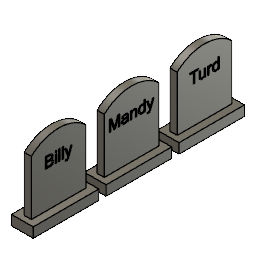
Nick Tomb Stones v2 (Autodesk Fusion 360 design; units mm, degrees)
Autodesk Fusion 360 part; units mm, degrees
note: some values were not read from the file. Set by a fixed rule: which face or edge a step refers to.
sketch "Sketch1" plane through (0, 0, 0) normal (1, 0, 0) x (0, 0, -1)
  line L0 (0, 0) -> (30, 0)
  line L1 (30, 0) -> (30, 36)
  line L2 (30, 36) -> (0, 36)
  line L3 (0, 36) -> (0, 0)
  line L4 (0, 36) -> (0, 30)
  line L5 (30, 36) -> (30, 30)
  arc A0 (30, 30) -> (0, 30) centre (15, 14.25) ccw
  dimension "d1" = 30
  dimension "d2" = 36
  dimension "d3" = 6
  dimension "d4" = 6
  constraint horizontal L0
  constraint vertical L1
  constraint horizontal L2
  constraint vertical L3
  constraint coincident L0.start L3.end
  constraint perpendicular L2 L4
  constraint perpendicular L2 L5
  constraint tangent L2 A0
  measures "d1" distance of L0.start L0.end
  measures "d2" distance of L0.start L2.end
  measures "d3" distance of L2.end L4.end
  measures "d4" distance of L1.end L5.end
extrude "Extrude1" add sketch "Sketch1" along normal blind 4 contours L0 L1 L3 A0 makes body 1
sketch "Sketch2" plane through (0, 0, 0) normal (0, -1, 0) x (1, 0, 0)
  line L0 (0, 0) -> (0, -30)
  line L1 (0, -30) -> (4, -30)
  line L2 (4, -30) -> (4, 0)
  line L3 (4, 0) -> (0, 0)
  line L4 (4, -15) -> (4, 3)
  line L5 (2, 0) -> (8, 0)
  line L6 (8, 3) -> (-4, 3)
  line L7 (-4, 3) -> (-4, -33)
  line L8 (-4, -33) -> (8, -33)
  line L9 (8, -33) -> (8, 3)
  dimension "d7" = 18
  dimension "d8" = 6
  dimension "d9" = 12
  dimension "d10" = 36
  constraint midpoint L2 L4.start
  constraint perpendicular L3 L4
  constraint midpoint L3 L5.start
  constraint perpendicular L0 L5
  constraint horizontal L6
  constraint vertical L7
  constraint horizontal L8
  constraint vertical L9
  measures "d7" distance of L4.start L4.end
  measures "d8" distance of L5.start L5.end
  measures "d9" distance of L6.start L6.end
  measures "d10" distance of L6.start L8.end
extrude "Extrude2" add sketch "Sketch2" along normal blind 6 separate body makes body 2
extrude "Extrude3" add 1 faces at (1.3333, 0, -10) along direction (0, -1, 0) blind 6 on bodies 1 bodies 1 2
sketch "Sketch3" plane through (4, 0, 0) normal (1, 0, 0) x (0, 0, -1)
  arc A0 (30, 30) -> (0, 30) centre (15, 14.25) ccw
  line L0 (0, 30) -> (0, 0)
  line L1 (0, 0) -> (30, 0)
  line L2 (30, 0) -> (30, 30)
  line L3 (0, 30) -> (2, 30)
  line L4 (2, 30) -> (2, 28)
  line L5 (2, 28) -> (0, 28)
  line L6 (0, 28) -> (0, 30)
  line L7 (2, 28) -> (28, 28)
  line L8 (28, 28) -> (28, 18)
  line L9 (28, 18) -> (2, 18)
  line L10 (2, 18) -> (2, 28)
  line L11 (2, 18) -> (28, 18) construction
  line L12 (28, 18) -> (28, 28) construction
  line L13 (28, 28) -> (2, 28) construction
  line L14 (2, 28) -> (2, 18) construction
  dimension "d15" = 2
  dimension "d16" = 2
  dimension "d17" = 26
  dimension "d18" = 10
  dimension "d19" = 6
  text T0 "Billy" font "Arial" height 6 align centre middle in box 26 x 10 at (2, 18) x (1, 0) y (0, 1) spacing 1 kerned
  constraint horizontal L3
  constraint vertical L4
  constraint horizontal L5
  constraint vertical L6
  constraint coincident A0.end L0.start
  constraint horizontal L7
  constraint vertical L8
  constraint horizontal L9
  constraint vertical L10
  constraint coincident L8.end
  constraint coincident L4.end
  measures "d15" distance of A0.end L3.end
  measures "d16" distance of A0.end L5.end
  measures "d17" distance of L4.end L7.end
  measures "d18" distance of L4.end L9.end
extrude "Extrude4" cut sketch "Sketch3" against normal blind 1 text T0 bodies 1
sketch "Sketch4" plane through (0, -6, 0) normal (0, -1, 0) x (1, 0, 0)
  line L0 (8, -33) -> (8, 3)
  line L1 (8, 3) -> (-4, 3)
  line L2 (-4, 3) -> (-4, -33)
  line L3 (-4, -33) -> (8, -33)
  line L4 (2, 3) -> (2, -33)
  line L5 (6.75, -12.2576) -> (2, -9.5152)
  line L6 (2, -9.5152) -> (-2.75, -12.2576)
  line L7 (-2.75, -12.2576) -> (-2.75, -17.7424)
  line L8 (-2.75, -17.7424) -> (2, -20.4848)
  line L9 (2, -20.4848) -> (6.75, -17.7424)
  line L10 (6.75, -17.7424) -> (6.75, -12.2576)
  point P0 (2, -15)
  dimension "d22" = 4.75
  constraint midpoint L1 L4.start
  constraint midpoint L3 L4.end
  constraint midpoint L4 P0
  measures "d22" distance of P0 L10
extrude "Extrude5" cut sketch "Sketch4" against normal blind 3.3 contours L4 L6 L7 L8 | L4 L5 L9 L10 bodies 1
sketch "Sketch5" plane through (0, -6, 0) normal (0, -1, 0) x (1, 0, 0)
  line L0 (2, -9.5152) -> (6.75, -12.2576)
  line L1 (6.75, -12.2576) -> (6.75, -17.7424)
  line L2 (6.75, -17.7424) -> (2, -20.4848)
  line L3 (2, -20.4848) -> (-2.75, -17.7424)
  line L4 (-2.75, -17.7424) -> (-2.75, -12.2576)
  line L5 (-2.75, -12.2576) -> (2, -9.5152)
  line L6 (8, -33) -> (8, 3)
  line L7 (8, 3) -> (-4, 3)
  line L8 (-4, 3) -> (-4, -33)
  line L9 (-4, -33) -> (8, -33)
  line L10 (2, -9.5152) -> (2, 3)
  line L11 (2, -20.4848) -> (2, -33)
  line L12 (4.7424, -31.4924) -> (7.4848, -26.7424)
  line L13 (7.4848, -26.7424) -> (4.7424, -21.9924)
  line L14 (4.7424, -21.9924) -> (-0.7424, -21.9924)
  line L15 (-0.7424, -21.9924) -> (-3.4848, -26.7424)
  line L16 (-3.4848, -26.7424) -> (-0.7424, -31.4924)
  line L17 (-0.7424, -31.4924) -> (4.7424, -31.4924)
  line L18 (4.7424, -8.0076) -> (7.4848, -3.2576)
  line L19 (7.4848, -3.2576) -> (4.7424, 1.4924)
  line L20 (4.7424, 1.4924) -> (-0.7424, 1.4924)
  line L21 (-0.7424, 1.4924) -> (-3.4848, -3.2576)
  line L22 (-3.4848, -3.2576) -> (-0.7424, -8.0076)
  line L23 (-0.7424, -8.0076) -> (4.7424, -8.0076)
  point P0 (2, -26.7424)
  point P1 (2, -3.2576)
  dimension "d25" = 4.75
  dimension "d26" = 4.75
  constraint coincident L0.start L5.end
  constraint midpoint L7 L10.end
  constraint coincident L2.end L3.start
  constraint midpoint L9 L11.end
  constraint midpoint L11 P0
  constraint midpoint L10 P1
  measures "d25" distance of P0 L17
  measures "d26" distance of P1 L23
extrude "Extrude6" cut sketch "Sketch5" against normal blind 3.3 contours L10 L20 L21 L22 L23 | L10 L18 L19 L20 L23 | L11 L12 L13 L14 L17 | L11 L14 L15 L16 L17 bodies 1
chamfer "Chamfer1" distance 0.5 angle 45 21 edges at (8, -6, -15) (2, -6, 3) (-4, -6, -15) (2, -6, -33) (6.1136, -6, -24.3674) (6.1136, -6, -29.1174) (2, -6, -31.4924) (-2.1136, -6, -29.1174) (-2.1136, -6, -24.3674) (-0.375, -6, -19.1136) (4.375, -6, -19.1136) (6.75, -6, -15) (4.375, -6, -10.8864) (-0.375, -6, -10.8864) (-2.75, -6, -15) (-2.1136, -6, -5.6326) (2, -6, -8.0076) (6.1136, -6, -5.6326) (6.1136, -6, -0.8826) (2, -6, 1.4924) (-2.1136, -6, -0.8826) on bodies 1
extrude "Extrude7" cut 3 faces at (1.0859, -2.7, -28.3257) (3.5833, -2.7, -15.9141) (1.0859, -2.7, -4.8409) along direction (0, 1, 0) blind 0.5 on bodies 1 bodies 1
copy_body "CopyPasteBodies1" bodies 1 makes body 3
move_body "Move1" bodies 3 to x (1, 0, 0) y (0, 1, 0) z (0, 0, 1) at (0, 0, -40)
extrude "Extrude8" add 6 faces at (3, 22.9236, -47.9243) (3, 21.4488, -53.6842) (3, 25.4352, -53.6842) (3, 22, -55.5259) (3, 22, -57.3881) (3, 22.0559, -59.4741) along direction (1, 0, 0) blind 1 on bodies 3 bodies 3
copy_body "CopyPasteBodies2" bodies 3 makes body 4
move_body "Move2" bodies 4 to x (1, 0, 0) y (0, 1, 0) z (0, 0, 1) at (0, 0, -40)
sketch "Sketch6" plane through (4, 0, 0) normal (1, 0, 0) x (0, 0, -1)
  arc A0 (70, 30) -> (40, 30) centre (55, 14.25) ccw
  line L0 (40, 30) -> (40, 0)
  line L1 (40, 0) -> (70, 0)
  line L2 (70, 0) -> (70, 30)
  line L3 (40, 30) -> (42, 30)
  line L4 (42, 30) -> (42, 28)
  line L5 (42, 28) -> (40, 28)
  line L6 (40, 28) -> (40, 30)
  line L7 (42, 28) -> (68, 28)
  line L8 (68, 28) -> (68, 18)
  line L9 (68, 18) -> (42, 18)
  line L10 (42, 18) -> (42, 28)
  line L11 (42, 18) -> (68, 18) construction
  line L12 (68, 18) -> (68, 28) construction
  line L13 (68, 28) -> (42, 28) construction
  line L14 (42, 28) -> (42, 18) construction
  dimension "d34" = 2
  dimension "d35" = 2
  dimension "d36" = 26
  dimension "d37" = 10
  dimension "d38" = 6
  text T0 "Mandy" font "Arial" height 6 align centre middle in box 26 x 10 at (42, 18) x (1, 0) y (0, 1) spacing 1 kerned
  constraint horizontal L3
  constraint vertical L4
  constraint horizontal L5
  constraint vertical L6
  constraint coincident A0.end L0.start
  constraint horizontal L7
  constraint vertical L8
  constraint horizontal L9
  constraint vertical L10
  constraint coincident L8.end
  constraint coincident L4.end
  measures "d34" distance of A0.end L3.end
  measures "d35" distance of A0.end L5.end
  measures "d36" distance of L4.end L7.end
  measures "d37" distance of L4.end L9.end
extrude "Extrude9" cut sketch "Sketch6" against normal blind 0.5 text T0 bodies 3
extrude "Extrude10" add 6 faces at (3, 22.9236, -7.9243) (3, 21.4488, -13.6842) (3, 25.4352, -13.6842) (3, 22, -15.5259) (3, 22, -17.3881) (3, 22.0559, -19.4741) along direction (1, 0, 0) blind 0.5 on bodies 1 bodies 1
sketch "Sketch7" plane through (4, 0, 0) normal (1, 0, 0) x (0, 0, -1)
  arc A0 (110, 30) -> (80, 30) centre (95, 14.25) ccw
  line L0 (80, 30) -> (80, 0)
  line L1 (80, 0) -> (110, 0)
  line L2 (110, 0) -> (110, 30)
  line L3 (80, 30) -> (82, 30)
  line L4 (82, 30) -> (82, 28)
  line L5 (82, 28) -> (80, 28)
  line L6 (80, 28) -> (80, 30)
  line L7 (82, 28) -> (108, 28)
  line L8 (108, 28) -> (108, 18)
  line L9 (108, 18) -> (82, 18)
  line L10 (82, 18) -> (82, 28)
  line L11 (82, 18) -> (108, 18) construction
  line L12 (108, 18) -> (108, 28) construction
  line L13 (108, 28) -> (82, 28) construction
  line L14 (82, 28) -> (82, 18) construction
  dimension "d43" = 2
  dimension "d44" = 2
  dimension "d45" = 26
  dimension "d46" = 10
  dimension "d47" = 6
  text T0 "Turd" font "Arial" height 6 align centre middle in box 26 x 10 at (82, 18) x (1, 0) y (0, 1) spacing 1 kerned
  constraint horizontal L3
  constraint vertical L4
  constraint horizontal L5
  constraint vertical L6
  constraint coincident A0.end L0.start
  constraint horizontal L7
  constraint vertical L8
  constraint horizontal L9
  constraint vertical L10
  constraint coincident L8.end
  constraint coincident L4.end
  measures "d43" distance of A0.end L3.end
  measures "d44" distance of A0.end L5.end
  measures "d45" distance of L4.end L7.end
  measures "d46" distance of L4.end L9.end
extrude "Extrude11" cut sketch "Sketch7" against normal blind 0.5 text T0 bodies 4
equation "d7 = ( 36 / 2 ) * 1 mm"
equation "d22 = ( 9.5 / 2 ) * 1 mm"
equation "d25 = ( 9.5 / 2 ) * 1 mm"
equation "d26 = ( 9.5 / 2 ) * 1 mm"
equation "d41 = 1.00 mm - 0.5 mm"
named bodies: "Billy", "Mandy", "Turd"
